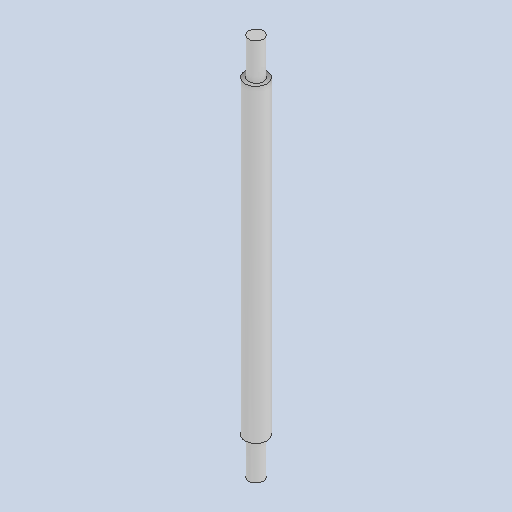
# Autodesk Inventor part: manipulo
Saved by Autodesk Inventor 2022.2 (Build 262287010, 287A)
## iProperties
Created: 2022-03-09
Part Number: manipulo
Material: Aluminum 6061-AHC
Document SubType Name: Modeling
Designer: Korch
Density: 2.7 g/cm^3
Appearance: Aluminum - Dark
Author: Korch
Autodesk Inventor part; units mm, degrees
ref_plane "YZ Plane" through (0, 0, 0) normal (1, 0, 0) x (0, 1, 0)
ref_plane "XZ Plane" through (0, 0, 0) normal (0, 1, 0) x (-1, 0, 0)
ref_plane "XY Plane" through (0, 0, 0) normal (0, 0, 1) x (1, 0, 0)
sketch "Sketch1" plane through (0, 0, 0) normal (0, 0, 1) x (1, 0, 0)
  line L0 (0, 0) -> (2, 0)
  line L1 (2, 0) -> (2, 10)
  line L2 (2, 10) -> (3, 10)
  line L3 (3, 10) -> (3, 94)
  line L4 (3, 94) -> (2, 94)
  line L5 (2, 94) -> (2, 104)
  line L6 (2, 104) -> (0, 104)
  line L7 (0, 104) -> (0, 0)
  dimension "d0" = 2
  dimension "d1" = 10
  dimension "d2" = 1
  dimension "d3" = 84
  dimension "d4" = 1
  dimension "d5" = 10
  constraints: 16 end point, 5 perpendicular, 2 point on line, 1 horizontal
  measures "d0" distance of L0.start L0.end
  measures "d1" distance of L0.end L1.end
  measures "d2" distance of L1.end L2.end
  measures "d3" distance of L2.end L3.end
  measures "d4" distance of L3.end L4.end
  measures "d5" distance of L4.end L5.end
revolve "Revolution1" add sketch "Sketch1" angle 360 about axis through (0, 104, 0) along (0, -1, 0)
body "Solid1"
